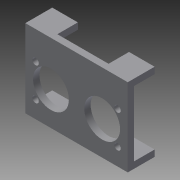
# Autodesk Inventor part: ping_bracket
Saved by Autodesk Inventor 2015 (Build 190159000, 159)
## iProperties
Created: 2014-10-29
Part Number: ping_bracket
Material: Generic
Document SubType Name: Modeling
Designer: Colin
Density: 1 g/cm^3
Appearance: Default
Author: Colin
Autodesk Inventor part; units mm, degrees
ref_plane "YZ Plane" through (0, 0, 0) normal (1, 0, 0) x (0, 1, 0)
ref_plane "XZ Plane" through (0, 0, 0) normal (0, 1, 0) x (-1, 0, 0)
ref_plane "XY Plane" through (0, 0, 0) normal (0, 0, 1) x (1, 0, 0)
sketch "Sketch1" plane through (0, 0, 0) normal (1, 0, 0) x (0, 1, 0)
  line L0 (0, 0) -> (35.56, 0)
  line L1 (35.56, -3.175) -> (3.175, -3.175)
  line L2 (3.175, -3.175) -> (3.175, -13.335)
  line L3 (3.175, -13.335) -> (0, -13.335)
  line L4 (0, -13.335) -> (0, 0)
  line L5 (35.56, 0) -> (38.735, 0)
  line L6 (38.735, 0) -> (38.735, -13.335)
  line L7 (38.735, -13.335) -> (35.56, -13.335)
  line L8 (35.56, -13.335) -> (35.56, -3.175)
  dimension "d0" = 3.175
  dimension "d1" = 35.56
  dimension "d33" = 13.335
  dimension "d34" = 3.175
  dimension "d48" = 90
  dimension "d49" = 13.335
  dimension "d50" = 3.175
  dimension "d51" = 10.16
  constraints: 18 end point, 4 perpendicular, 2 horizontal, 2 parallel
  measures "d0" distance of L2.end L3.end
  measures "d1" distance of L0.start L0.end
  measures "d33" distance of L3.end L0.start
  measures "d34" distance of L0.end L1.start
  measures "d48" angle of L0 L4
  measures "d49" distance of L5.end L6.end
  measures "d50" distance of L6.end L7.end
  measures "d51" distance of L1.end L2.end
extrude "Extrusion1" add sketch "Sketch1" along normal blind 50.8
sketch "Sketch3" plane through (0, 0, 0) normal (0, 0, 1) x (1, 0, 0)
  line L0 (0, 35.56) -> (50.8, 35.56) projected
  line L1 (25.4, 35.56) -> (25.4, 3.175) construction
  line L2 (0, 3.175) -> (50.8, 3.175) projected
  circle A0 centre (12.7, 16.637) radius 8.89
  circle A1 centre (38.1, 16.637) radius 8.89
  line L3 (0, 0) -> (0, 35.56) projected
  line L4 (0, 27.305) -> (50.8, 27.305) construction
  line L5 (0, 5.969) -> (52.4314, 5.969) construction
  line L6 (2.54, 27.305) -> (2.54, 5.969) construction
  line L7 (48.26, 27.305) -> (48.26, 5.969) construction
  circle A2 centre (5.08, 8.509) radius 1.5875
  circle A3 centre (45.72, 24.765) radius 1.5875
  circle A4 centre (5.08, 24.765) radius 1.5875
  circle A5 centre (45.72, 8.509) radius 1.5875
  dimension "d7" = 17.78
  dimension "d8" = 12.7
  dimension "d13" = 10.668
  dimension "d14" = 10.668
  dimension "d15" = 10.16
  dimension "d16" = 10.16
  dimension "d17" = 3.175
  dimension "d19" = 2.54
  dimension "d20" = 3.175
  dimension "d21" = 2.54
  dimension "d25" = 2.54
  dimension "d26" = 2.54
  dimension "d38" = 3.175
  dimension "d39" = 2.54
  dimension "d40" = 2.54
  dimension "d41" = 3.175
  dimension "d42" = 2.54
  dimension "d43" = 2.54
  dimension "d53" = 2.794
  constraints: 10 end point, 6 centre point, 6 point on line, 2 horizontal, 2 midpoint, 2 perpendicular, 1 symmetric about line, 1 other
  measures "d7" diameter of A0
  measures "d8" distance from line of L1 A0.centre
  measures "d13" distance from line of A1.centre L5
  measures "d14" distance from line of A1.centre L4
  measures "d15" distance from line of A0.centre L6
  measures "d16" distance from line of A1.centre L7
  measures "d17" diameter of A2
  measures "d19" distance from line of L6 A2.centre
  measures "d20" diameter of A3
  measures "d21" distance from line of L7 A3.centre
  measures "d25" distance from line of L5 A2.centre
  measures "d26" distance from line of L4 A3.centre
  measures "d38" diameter of A4
  measures "d39" distance from line of L4 A4.centre
  measures "d40" distance from line of L6 A4.centre
  measures "d41" diameter of A5
  measures "d42" distance from line of L5 A5.centre
  measures "d43" distance from line of L7 A5.centre
  measures "d53" distance between parallel lines of L2 L5
extrude "Extrusion2" cut sketch "Sketch3" against normal through all
sketch "Sketch5" plane through (0, 38.735, 0) normal (0, 1, 0) x (1, 0, 0)
  line L0 (0, 0) -> (50.8, 0) construction
  line L1 (0, 3.175) -> (50.8, 3.175) construction
  line L2 (12.7, 3.175) -> (12.7, 13.335)
  line L3 (0, 13.335) -> (50.8, 13.335) projected
  line L4 (38.1, 3.175) -> (38.1, 13.335)
  line L5 (0, 0) -> (0, 13.335) projected
  line L6 (12.7, 3.175) -> (38.1, 3.175)
  line L7 (12.7, 13.335) -> (38.1, 13.335)
  dimension "d44" = 25.4
  dimension "d45" = 12.7
  constraints: 8 end point, 4 point on line, 2 collinear, 1 perpendicular, 1 vertical
  measures "d44" distance between parallel lines of L2 L4
  measures "d45" distance between parallel lines of L5 L2
extrude "Extrusion4" cut sketch "Sketch5" against normal through all
equation "\"d49\" = d33"
equation "\"d50\" = d0"
body "Solid1"
